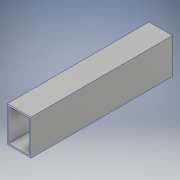
# Autodesk Inventor part: 2x2x1_8_rectangularTubing
Saved by Autodesk Inventor 2018.2 (Build 222227000, 227)
## iProperties
Created: 2018-01-09
Part Number: 2x2x1_8_rectangularTubing
Material: Aluminum 6061
Document SubType Name: Modeling
Designer: steele
Density: 2.7 g/cm^3
Appearance: Aluminum - Flat
Author: steele
Autodesk Inventor part; units mm, degrees
ref_plane "YZ Plane" through (0, 0, 0) normal (1, 0, 0) x (0, 1, 0)
ref_plane "XZ Plane" through (0, 0, 0) normal (0, 1, 0) x (-1, 0, 0)
ref_plane "XY Plane" through (0, 0, 0) normal (0, 0, 1) x (1, 0, 0)
sketch "Sketch1" plane through (0, 0, 0) normal (0, 0, 1) x (1, 0, 0)
  line L0 (-25.4, -38.1) -> (25.4, -38.1)
  line L1 (25.4, -38.1) -> (25.4, 38.1)
  line L2 (25.4, 38.1) -> (-25.4, 38.1)
  line L3 (-25.4, 38.1) -> (-25.4, -38.1)
  line L4 (-25.4, -38.1) -> (25.4, 38.1) construction
  line L5 (25.4, -38.1) -> (-25.4, 38.1) construction
  line L6 (-22.225, -34.925) -> (22.225, -34.925)
  line L7 (22.225, -34.925) -> (22.225, 34.925)
  line L8 (22.225, 34.925) -> (-22.225, 34.925)
  line L9 (-22.225, 34.925) -> (-22.225, -34.925)
  line L10 (-22.225, -34.925) -> (22.225, 34.925) construction
  line L11 (22.225, -34.925) -> (-22.225, 34.925) construction
  point P0 (0, 0)
  dimension "d0" = 50.8
  dimension "d1" = 76.2
  dimension "d2" = 3.175
  dimension "d3" = 3.175
  constraints: 24 end point, 5 parallel, 4 midpoint, 2 perpendicular, 1 horizontal
  measures "d0" distance of L0.start L0.end
  measures "d1" distance of L1.end L0.end
  measures "d2" distance between parallel lines of L6 L0
  measures "d3" distance between parallel lines of L3 L9
extrude "Extrusion1" add sketch "Sketch1" against normal blind 304.8
body "Solid1"
